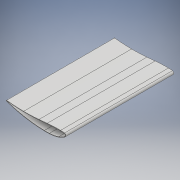
# Autodesk Inventor part: GFRP_sf
Saved by Autodesk Inventor 2018.2 (Build 222227000, 227)
## iProperties
Created: 2018-04-22
Part Number: GFRP_sf
Material: 一般
Document SubType Name: Modeling
Designer: ku_sk
Density: 1 g/cm^3
Appearance: 既定
Author: ku_sk
Autodesk Inventor part; units mm, degrees
ref_plane "YZ Plane" through (0, 0, 0) normal (1, 0, 0) x (0, 1, 0)
ref_plane "XZ Plane" through (0, 0, 0) normal (0, 1, 0) x (-1, 0, 0)
ref_plane "XY Plane" through (0, 0, 0) normal (0, 0, 1) x (1, 0, 0)
sketch "スケッチ1" plane through (0, 0, 0) normal (0, 1, 0) x (-1, 0, 0)
  arc A0 (41.4271, -13.9695) -> (120.4366, 0.3359) centre (36.8758, 236.5065) ccw projected
  arc A1 (30.7593, -13.8476) -> (41.4271, -13.9695) centre (38.1525, 166.2425) ccw projected
  arc A2 (11.3224, -10.3926) -> (30.7593, -13.8476) centre (33.77, 59.49) ccw projected
  arc A3 (0.21, -4.9345) -> (11.3224, -10.3926) centre (24.3575, 30.1875) ccw projected
  arc A4 (-2.7782, -2.0329) -> (0.21, -4.9345) centre (7.25, 5.305) ccw projected
  arc A5 (-0.6081, 3.3884) -> (-2.7782, -2.0329) centre (0, 0) ccw projected
  arc A6 (7.6216, 4.1344) -> (-0.6081, 3.3884) centre (7.775, -43.32) ccw projected
  arc A7 (35.4685, 2.8931) -> (7.6216, 4.1344) centre (8.565, -287.665) ccw projected
  arc A8 (35.4685, 2.8931) -> (52.5963, 1.3351) centre (526.9475, 5310.875) ccw projected
  arc A9 (52.5963, 1.3351) -> (84.6296, -0.0095) centre (82.86, 340.0849) ccw projected
  arc A10 (84.6296, -0.0095) -> (119.9797, 2.271) centre (83.0725, 299.245) ccw projected
  arc A11 (120.4366, 0.3359) -> (119.9797, 2.271) centre (120.103, 1.2786) ccw projected
  circle A12 centre (10, -2) radius 3 projected
  circle A13 centre (85, -5) radius 3 projected
extrude "押し出し1" add sketch "スケッチ1" along normal mid plane 225 contours A1 A2 A3 A4 A5 A6 A7 A8 A9 A10 A11 A0 | A12 | A13
shell "シェル1" thickness 1 removed faces 2 at (-51.857, -112.5, -8.4758) at (-51.857, 112.5, -8.4758)
